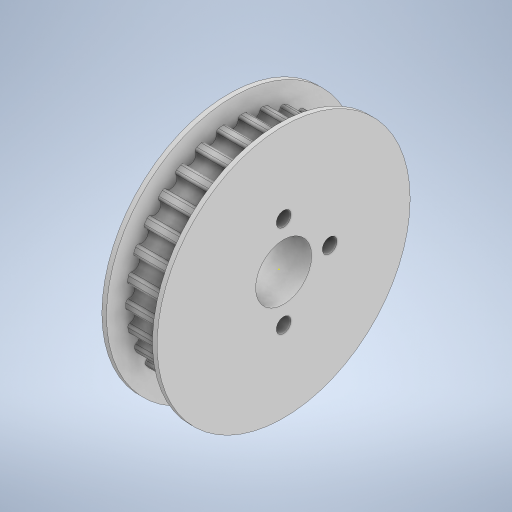
# Autodesk Inventor part: 射出_プーリ30完成
Saved by Autodesk Inventor 2023 (Build 270158000, 158)
## iProperties
Created: 2022-04-30
Part Number: 射出_プーリ30完成
Material: 一般
Document SubType Name: Modeling
Designer: yuta
Density: 1 g/cm^3
Appearance: 既定
Author: yuta
Autodesk Inventor part; units mm, degrees
ref_plane "YZ Plane" through (0, 0, 0) normal (1, 0, 0) x (0, 1, 0)
ref_plane "XZ Plane" through (0, 0, 0) normal (0, 1, 0) x (-1, 0, 0)
ref_plane "XY Plane" through (0, 0, 0) normal (0, 0, 1) x (1, 0, 0)
sketch "スケッチ1" plane through (0, 0, 0) normal (1, 0, 0) x (0, 1, 0)
  circle A0 centre (0, 0) radius 23.875 construction
  arc A1 (20.3373, 11.3774) -> (19.8134, 12.2671) centre (0, 0) ccw construction
  circle A2 centre (0, 0) radius 21.3735 construction
  arc A3 (20.1105, 10.6675) -> (20.3373, 11.3774) centre (19.8922, 11.1284) ccw
  line L0 (0, 0) -> (17.1826, 12.7115)
  arc A4 (17.1826, 12.7115) -> (19.0825, 12.4131) centre (18.284, 13.5263) ccw
  arc A5 (19.8134, 12.2671) -> (19.0825, 12.4131) centre (19.3798, 11.9987) ccw
  arc A6 (20.1105, 10.6675) -> (19.45, 8.8613) centre (20.6967, 9.4293) ccw
  line L1 (19.45, 8.8613) -> (0, 0)
  arc A7 (20.3373, 11.3774) -> (19.8134, 12.2671) centre (0, 0) ccw
  arc A8 (19.8134, 12.2671) -> (20.3373, 11.3774) centre (0, 0) ccw construction
  dimension "d0" = 47.75
  dimension "d2" = 42.747
  dimension "d6" = 1.02
  constraints: 14 point on circle, 9 centre point, 4 coincident, 4 end point, 1 concentric, 1 tangent
  measures "d0" diameter of A0
  measures "d2" diameter of A2
  measures "d6" diameter of A3
extrude "押し出し1" add sketch "スケッチ1" against normal blind 10
pattern_circular "円形状パターン1" count 30 over 360 about axis through (-10, 0, 0) along (1, 0, 0) of "押し出し1"
sketch "スケッチ2" plane through (-10, 0, 0) normal (-1, 0, 0) x (0, 0, 1)
  circle A0 centre (0, 0) radius 27.5
  dimension "d13" = 55
  constraints: 1 centre point, 1 coincident
  measures "d13" diameter of A0
extrude "押し出し2" add sketch "スケッチ2" along normal blind 1
sketch "スケッチ3" plane through (-11, 0, 0) normal (-1, 0, 0) x (0, 0, 1)
  circle A0 centre (0, 0) radius 6.1
  circle A1 centre (0, 10) radius 1.6
  circle A2 centre (-10, 0) radius 1.6
  circle A3 centre (0, -10) radius 1.6
  dimension "d16" = 12.2
  dimension "d17" = 3.2
  dimension "d18" = 3.2
  dimension "d19" = 3.2
  dimension "d20" = 10
  dimension "d21" = 10
  dimension "d22" = 10
  constraints: 4 centre point, 1 coincident
  measures "d16" diameter of A0
  measures "d17" diameter of A1
  measures "d18" diameter of A2
  measures "d19" diameter of A3
  measures "d20" distance of point (0, 0) A1.centre
  measures "d21" distance of point (0, 0) A2.centre
  measures "d22" distance of point (0, 0) A3.centre
extrude "押し出し3" cut sketch "スケッチ3" against normal blind 17
sketch "スケッチ4" plane through (0, 0, 0) normal (1, 0, 0) x (0, 0, -1)
  point P0 (0, 0)
sketch "スケッチ5" plane through (0, 0, 0) normal (1, 0, 0) x (0, 0, -1)
  circle A0 centre (0, 0) radius 27.5
  constraints: 1 centre point, 1 coincident
extrude "押し出し4" add sketch "スケッチ5" along normal blind 1
sketch "スケッチ6" plane through (1, 0, 0) normal (1, 0, 0) x (0, 0, -1)
  circle A0 centre (0, 0) radius 6.1
  circle A1 centre (0, 10) radius 1.6 projected
  circle A2 centre (0, 10) radius 1.6
  circle A3 centre (0, -10) radius 1.6 projected
  circle A4 centre (0, -10) radius 1.6
  circle A5 centre (10, 0) radius 1.6 projected
  circle A6 centre (10, 0) radius 1.6
  dimension "d27" = 12.2
  dimension "d28" = 3.2
  dimension "d29" = 3.2
  constraints: 4 centre point, 4 coincident
  measures "d27" diameter of A0
  measures "d28" diameter of A4
  measures "d29" diameter of A6
extrude "押し出し5" cut sketch "スケッチ6" against normal blind 17
